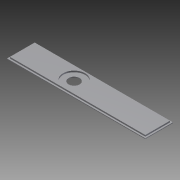
# Autodesk Inventor part: Tapa
Saved by Autodesk Inventor 2011 (Build 150239000, 239)
## iProperties
Created: 2014-08-04
Part Number: Tapa
Material: Por defecto
Document SubType Name: Chapa
Designer: amatiasq
Density: 1 g/cm^3
Sheet Metal Rule: Por defecto_mm
Author: amatiasq
Autodesk Inventor part; units mm, degrees
ref_plane "YZ Plane" through (0, 0, 0) normal (1, 0, 0) x (0, 1, 0)
ref_plane "XZ Plane" through (0, 0, 0) normal (0, 1, 0) x (-1, 0, 0)
ref_plane "XY Plane" through (0, 0, 0) normal (0, 0, 1) x (1, 0, 0)
sketch "Boceto1" plane through (0, 0, 0) normal (0, 0, 1) x (1, 0, 0)
  line L0 (0, 0) -> (200, 0)
  line L1 (200, 0) -> (200, 40)
  line L2 (200, 40) -> (0, 40)
  line L3 (0, 40) -> (0, 0)
  circle A0 centre (77, 20) radius 8
  dimension "d0" = 200
  dimension "d1" = 40
  dimension "d2" = 16
  constraints: 8 end point, 2 parallel, 1 centre point, 1 horizontal, 1 perpendicular
  measures "d0" distance of L2.end L1.end
  measures "d1" distance of L1.end L0.end
  measures "d2" diameter of A0
extrude "Extrusión1" add sketch "Boceto1" along normal blind 1
sketch "Boceto2" plane through (0, 0, 1) normal (0, 0, 1) x (1, 0, 0)
  circle A0 centre (77, 20) radius 8 projected
  line L0 (2.1, 2.1) -> (197.9, 2.1)
  line L1 (197.9, 2.1) -> (197.9, 37.9)
  line L2 (197.9, 37.9) -> (2.1, 37.9)
  line L3 (2.1, 37.9) -> (2.1, 2.1)
  circle A1 centre (77, 20) radius 16
  dimension "d5" = 195.8
  dimension "d6" = 35.8
  dimension "d7" = 32
  constraints: 8 end point, 2 parallel, 1 centre point, 1 coincident, 1 horizontal, 1 perpendicular
  measures "d5" distance of L2.end L1.end
  measures "d6" distance of L1.end L0.end
  measures "d7" diameter of A1
extrude "Extrusión2" add sketch "Boceto2" along normal blind 2 contours L3 L2 L1 L0
equation "\"Radio_pliegue\" = Grosor"
equation "\"Anchura_desahogo_plegado\" = Grosor"
equation "\"Profundidad_desahogo_plegado\" = 0.5 * Grosor"
equation "\"Tamaño_destalonado\" = 4 * Grosor"
equation "\"Remanente_mínimo\" = 2 * Grosor"
equation "\"Radiodetransición\" = Radio_pliegue"
equation "\"Tamaño_de_radio_de_Jacobi\" = Radio_pliegue"
equation "\"TamañoSeparación\" = Grosor"
equation "\"Grosor\" = 0.5"
